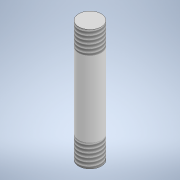
# Autodesk Inventor part: M3_16_shaft
Saved by Autodesk Inventor 2020.3 (Build 243373000, 373)
## iProperties
Created: 2021-03-23
Part Number: M3_16_shaft
Material: Ogólny
Document SubType Name: Modeling
Designer: patry
Density: 1 g/cm^3
Appearance: Domyślna
Author: patry
Autodesk Inventor part; units mm, degrees
ref_plane "YZ Plane" through (0, 0, 0) normal (1, 0, 0) x (0, 1, 0)
ref_plane "XZ Plane" through (0, 0, 0) normal (0, 1, 0) x (-1, 0, 0)
ref_plane "XY Plane" through (0, 0, 0) normal (0, 0, 1) x (1, 0, 0)
sketch "Szkic1" plane through (0, 0, 0) normal (0, 1, 0) x (-1, 0, 0)
  circle A0 centre (0, 0) radius 3.5
  line L0 (0.7217, 1.25) -> (1.4434, 0)
  line L1 (1.4434, 0) -> (0.7217, -1.25)
  line L2 (0.7217, -1.25) -> (-0.7217, -1.25)
  line L3 (-0.7217, -1.25) -> (-1.4434, 0)
  line L4 (-1.4434, 0) -> (-0.7217, 1.25)
  line L5 (-0.7217, 1.25) -> (0.7217, 1.25)
  circle A1 centre (0, 0) radius 1.5
  dimension "d0" = 7
  dimension "d1" = 2.5
  dimension "d2" = 3
  constraints: 12 end point, 3 coincident, 2 centre point, 13 other
  measures "d0" diameter of A0
  measures "d1" distance between parallel lines of L2 L5
  measures "d2" diameter of A1
extrude "Wyciągnięcie proste4" add sketch "Szkic1" along normal blind 16 contours L0 L1 L2 L3 L4 L5 | A1
thread "Gwint2" size "M3x0.5" class "6g" standard "ANSI Metric M Profile" length 3
thread "Gwint3" size "M3x0.5" class "6g" standard "ANSI Metric M Profile" length 3
